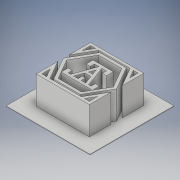
# Autodesk Inventor part: A_main
Saved by Autodesk Inventor 2019 (Build 230136000, 136)
## iProperties
Created: 2018-08-07
Part Number: A_main
Material: Generic
Document SubType Name: Modeling
Designer: Ge Shi
Density: 1 g/cm^3
Appearance: Default
Author: Ge Shi
Autodesk Inventor part; units mm, degrees
ref_plane "YZ Plane" through (0, 0, 0) normal (1, 0, 0) x (0, 1, 0)
ref_plane "XZ Plane" through (0, 0, 0) normal (0, 1, 0) x (-1, 0, 0)
ref_plane "XY Plane" through (0, 0, 0) normal (0, 0, 1) x (1, 0, 0)
sketch "Sketch1" plane through (0, 0, 0) normal (0, 1, 0) x (-1, 0, 0)
  line L0 (-10, 10) -> (10, 10)
  line L1 (10, 10) -> (10, -10)
  line L2 (10, -10) -> (-10, -10)
  line L3 (-10, -10) -> (-10, 10)
  line L4 (-10, 10) -> (10, -10) construction
  line L5 (10, 10) -> (-10, -10) construction
  line L6 (-9.5, 0) -> (-4.75, 8.2272)
  line L7 (-4.75, 8.2272) -> (4.75, 8.2272)
  line L8 (4.75, 8.2272) -> (9.5, 0)
  line L9 (9.5, 0) -> (4.75, -8.2272)
  line L10 (4.75, -8.2272) -> (-4.75, -8.2272)
  line L11 (-4.75, -8.2272) -> (-9.5, 0)
  line L12 (-8.3453, 0) -> (-4.1726, 7.2272)
  line L13 (-4.1726, 7.2272) -> (4.1726, 7.2272)
  line L14 (4.1726, 7.2272) -> (8.3453, 0)
  line L15 (8.3453, 0) -> (4.1726, -7.2272)
  line L16 (4.1726, -7.2272) -> (-4.1726, -7.2272)
  line L17 (-4.1726, -7.2272) -> (-8.3453, 0)
  line L18 (2.1284, -3.7272) -> (2.1284, -2.2272)
  line L19 (2.1284, -2.2272) -> (3.6284, -2.2272)
  line L20 (3.6284, -2.2272) -> (3.6284, -4.7272)
  line L21 (3.6284, -4.7272) -> (0, -4.7272)
  line L22 (0, -4.7272) -> (0, -2.2272)
  line L23 (0, -2.2272) -> (0.7279, -0.2272)
  line L24 (0.7279, -0.2272) -> (0, -0.2272)
  line L25 (0, -0.2272) -> (0, 0.7728)
  line L26 (0, 0.7728) -> (1.0919, 0.7728)
  line L27 (3.2314, 3.7272) -> (0.5182, -3.7272)
  line L28 (0.5182, -3.7272) -> (2.1284, -3.7272)
  line L29 (3.2314, 3.7272) -> (4.116, 3.7272)
  line L30 (4.116, 3.7272) -> (4.116, 2.2272)
  line L31 (4.116, 2.2272) -> (5.616, 2.2272)
  line L32 (5.616, 2.2272) -> (5.616, 4.7272)
  line L33 (5.616, 4.7272) -> (2.2598, 4.7272)
  line L34 (1.0919, 0.7728) -> (2.1673, 3.7272)
  line L35 (2.1673, 3.7272) -> (0.5571, 3.7272)
  line L36 (0.5571, 3.7272) -> (0.5571, 2.2272)
  line L37 (0.5571, 2.2272) -> (0, 2.2272)
  line L38 (0, 2.2272) -> (0, 4.7272)
  line L39 (0, 4.7272) -> (2.2598, 4.7272)
  line L40 (-2.1284, -3.7272) -> (-2.1284, -2.2272)
  line L41 (-2.1284, -2.2272) -> (-3.6284, -2.2272)
  line L42 (-3.6284, -2.2272) -> (-3.6284, -4.7272)
  line L43 (-3.6284, -4.7272) -> (0, -4.7272)
  line L44 (0, -2.2272) -> (-0.7279, -0.2272)
  line L45 (-0.7279, -0.2272) -> (0, -0.2272)
  line L46 (0, 0.7728) -> (-1.0919, 0.7728)
  line L47 (-3.2314, 3.7272) -> (-0.5182, -3.7272)
  line L48 (-0.5182, -3.7272) -> (-2.1284, -3.7272)
  line L49 (-3.2314, 3.7272) -> (-4.116, 3.7272)
  line L50 (-4.116, 3.7272) -> (-4.116, 2.2272)
  line L51 (-4.116, 2.2272) -> (-5.616, 2.2272)
  line L52 (-5.616, 2.2272) -> (-5.616, 4.7272)
  line L53 (-5.616, 4.7272) -> (-2.2598, 4.7272)
  line L54 (-1.0919, 0.7728) -> (-2.1673, 3.7272)
  line L55 (-2.1673, 3.7272) -> (-0.5571, 3.7272)
  line L56 (-0.5571, 3.7272) -> (-0.5571, 2.2272)
  line L57 (-0.5571, 2.2272) -> (0, 2.2272)
  line L58 (0, 4.7272) -> (-2.2598, 4.7272)
  line L59 (5.616, -8.7272) -> (9.5, -2)
  line L60 (9.5, -2) -> (9.5, -9.7272)
  line L61 (9.5, -9.7272) -> (0, -9.7272)
  line L62 (0, -9.7272) -> (0, -8.7272)
  line L63 (0, -8.7272) -> (5.616, -8.7272)
  line L64 (6.7707, -8.7272) -> (8.5, -8.7272)
  line L65 (8.5, -8.7272) -> (8.5, -5.7321)
  line L66 (8.5, -5.7321) -> (6.7707, -8.7272)
  line L67 (-5.616, -8.7272) -> (-9.5, -2)
  line L68 (-9.5, -2) -> (-9.5, -9.7272)
  line L69 (-9.5, -9.7272) -> (0, -9.7272)
  line L70 (0, -8.7272) -> (-5.616, -8.7272)
  line L71 (-6.7707, -8.7272) -> (-8.5, -8.7272)
  line L72 (-8.5, -8.7272) -> (-8.5, -5.7321)
  line L73 (-8.5, -5.7321) -> (-6.7707, -8.7272)
  line L74 (10, 0) -> (14.2645, 0) construction
  line L75 (-10, -10) -> (10, 10) construction
  line L76 (4.75, 8.2272) -> (-4.75, 8.2272)
  line L77 (5.616, 8.7272) -> (9.5, 2)
  line L78 (9.5, 2) -> (9.5, 9.7272)
  line L79 (9.5, 9.7272) -> (0, 9.7272)
  line L80 (0, 9.7272) -> (0, 8.7272)
  line L81 (0, 8.7272) -> (5.616, 8.7272)
  line L82 (6.7707, 8.7272) -> (8.5, 8.7272)
  line L83 (8.5, 8.7272) -> (8.5, 5.7321)
  line L84 (8.5, 5.7321) -> (6.7707, 8.7272)
  line L85 (-9.5, 9.7272) -> (0, 9.7272)
  line L86 (-6.7707, 8.7272) -> (-8.5, 8.7272)
  line L87 (-8.5, 5.7321) -> (-6.7707, 8.7272)
  line L88 (-8.5, 8.7272) -> (-8.5, 5.7321)
  line L89 (-9.5, 2) -> (-9.5, 9.7272)
  line L90 (-5.616, 8.7272) -> (-9.5, 2)
  line L91 (0, 8.7272) -> (-5.616, 8.7272)
  point P0 (0, 0)
  point P1 (0, 0)
  point P2 (0, 0)
  point P3 (0, -7.2272)
  dimension "d0" = 20
  dimension "d1" = 20
  dimension "d2" = 0.5
  dimension "d3" = 1
  dimension "d4" = 1.5
  dimension "d5" = 1
  dimension "d6" = 1.5
  dimension "d7" = 1
  dimension "d9" = 70
  dimension "d13" = 1.5
  dimension "d14" = 1.5
  dimension "d15" = 1
  dimension "d16" = 1
  dimension "d17" = 2
  dimension "d18" = 1
  dimension "d19" = 2.5
  dimension "d23" = 1
  dimension "d26" = 2.5
  dimension "d29" = 0.5
  dimension "d30" = 1
  dimension "d32" = 1
  dimension "d33" = 1
  dimension "d34" = 1
  constraints: 184 end point, 36 symmetric about line, 14 perpendicular, 13 point on line, 7 horizontal, 6 parallel, 4 coincident, 4 collinear, 4 midpoint, 2 vertical, 26 other
  measures "d0" distance of L1.end L2.end
  measures "d1" distance of L0.end L1.end
  measures "d2" distance from line of L1 L8.end
  measures "d3" distance between parallel lines of L11 L17
  measures "d4" distance between parallel lines of L20 L18
  measures "d5" distance between parallel lines of L21 L28
  measures "d6" distance between parallel lines of L28 L19
  measures "d7" distance between parallel lines of L27 L23
  measures "d9" angle of L28 L27
  measures "d13" distance of L30.end L31.end
  measures "d14" distance of L29.end L30.end
  measures "d15" distance between parallel lines of L29 L33
  measures "d16" distance from line of L27 L18.end
  measures "d17" distance from line of L22.end L24
  measures "d18" distance between parallel lines of L26 L24
  measures "d19" distance between parallel lines of L16 L21
  measures "d23" distance from line of L34 L36.end
  measures "d26" distance between parallel lines of L13 L33
  measures "d29" distance between parallel lines of L10 L63
  measures "d30" distance between parallel lines of L61 L63
  measures "d32" distance between parallel lines of L59 L66
  measures "d33" distance between parallel lines of L60 L65
  measures "d34" distance between parallel lines of L9 L59
extrude "Extrusion1" add sketch "Sketch1" along normal blind 10 contours L6 L7 L8 L9 L10 L11 | L53 L58 L38 L57 L56 L55 L54 L46 L25 L45 L44 L22 L43 L42 L41 L40 L48 L47 L49 L50 L51 L52 | L39 L33 L32 L31 L30 L29 L27 L28 L18 L19 L20 L21 L22 L23 L24 L25 L26 L34 L35 L36 L37 L38 | L59 L60 L61 L62 L63 | L62 L69 L68 L67 L70 | L81 L80 L79 L78 L77 | L91 L90 L89 L85 L80
sketch "Sketch2" plane through (0, 0, 0) normal (0, 1, 0) x (-1, 0, 0)
  line L0 (-15, 15) -> (15, 15)
  line L1 (15, 15) -> (15, -15)
  line L2 (15, -15) -> (-15, -15)
  line L3 (-15, -15) -> (-15, 15)
  line L4 (-15, 15) -> (15, -15) construction
  line L5 (15, 15) -> (-15, -15) construction
  point P0 (0, 0)
  dimension "d35" = 30
  dimension "d36" = 30
  constraints: 12 end point, 2 midpoint, 2 parallel, 1 horizontal, 1 perpendicular
  measures "d35" distance of L1.end L2.end
  measures "d36" distance of L0.end L1.end
extrude "Extrusion2" add sketch "Sketch2" against normal blind 0.2
equation "\"d2\" = mini"
equation "\"d3\" = 2 * mini"
equation "\"nozzleHead\" = 0.5"
equation "\"mini\" = nozzleHead"
body "Solid1"
